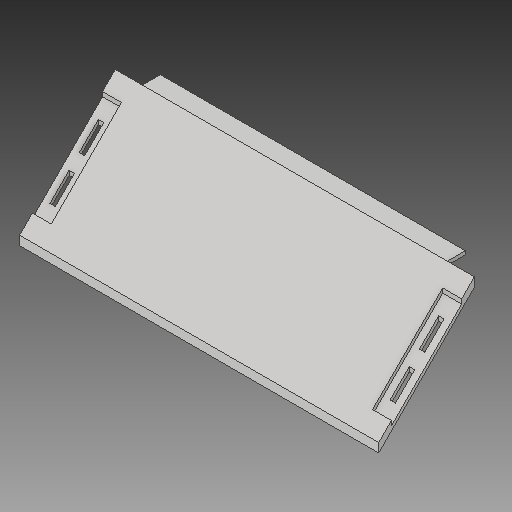
# Autodesk Inventor part: Roof Width Extension
Saved by Autodesk Inventor 2017 (Build 210142000, 142)
## iProperties
Created: 2018-03-29
Part Number: Roof Width Extension
Material: Generic
Document SubType Name: Modeling
Designer: Arjuna
Density: 1 g/cm^3
Appearance: Default
Author: Arjuna
Autodesk Inventor part; units mm, degrees
ref_plane "YZ Plane" through (0, 0, 0) normal (1, 0, 0) x (0, 1, 0)
ref_plane "XZ Plane" through (0, 0, 0) normal (0, 1, 0) x (-1, 0, 0)
ref_plane "XY Plane" through (0, 0, 0) normal (0, 0, 1) x (1, 0, 0)
sketch "Sketch2" plane through (0, 0, 0) normal (0, 0, 1) x (1, 0, 0)
  line L0 (-99.5, 2.5) -> (99.5, 2.5)
  line L1 (99.5, 2.5) -> (99.5, -2.5)
  line L2 (99.5, -2.5) -> (-99.5, -2.5)
  line L3 (-99.5, -2.5) -> (-99.5, 2.5)
  point P0 (0, 0)
  dimension "d1" = 199
  dimension "d2" = 5
  dimension "d3" = 2.5
  dimension "d4" = 99.5
  constraints: 8 end point, 2 parallel, 1 horizontal, 1 perpendicular
  measures "d1" distance of L1.end L2.end
  measures "d2" distance of L2.end L0.start
  measures "d3" vertical distance of point (0, 0) L0.start
  measures "d4" distance from line of point (0, 0) L3
sketch "Sketch3" plane through (0, 0, 0) normal (1, 0, 0) x (0, 1, 0)
  line L0 (0, 0) -> (-53.033, 53.033)
  line L1 (0, -0.5221) -> (1.6531, -0.5221)
  dimension "d5" = 75
  dimension "d6" = 45
  constraints: 4 end point, 1 horizontal
  measures "d5" distance of L0.start L0.end
  measures "d6" angle of L1 L0
sweep "Sweep1" add profiles "Sketch2" path "Sketch3" path curves L0
sketch "Sketch4" plane through (-99.5, 2.5, 0) normal (0, 0.7071068, 0.7071068) x (1, 0, 0)
  line L0 (0, 0) -> (199, 0) projected
  line L1 (0, 0) -> (0, -75) projected
  line L2 (199, -75) -> (0, -75) projected
  line L3 (199, 0) -> (199, -75) projected
  line L4 (199, 0) -> (199, -75)
  line L5 (199, 0) -> (274, -75)
  line L6 (274, -75) -> (199, -75)
  point P0 (99.5, -1.7678)
  dimension "d9" = 45
  constraints: 6 end point, 2 collinear
  measures "d9" angle of L5 L3
sketch "Sketch5" plane through (99.5, -2.5, 0) normal (1, 0, 0) x (0, 0, -1)
  line L0 (0, 5) -> (0, 0) projected
  line L1 (0, 5) -> (-53.033, -48.033) projected
  line L2 (-53.033, -53.033) -> (-53.033, -48.033) projected
  line L3 (0, 0) -> (-53.033, -53.033) projected
  line L4 (-26.5165, -21.5165) -> (-26.5165, -26.5165)
  point P0 (0, 2.5)
  constraints: 2 end point, 2 midpoint
sweep "Sweep2" [suppressed]
mirror "Mirror1" [suppressed]
sketch "Sketch6" plane through (99.5, 2.5, 0) normal (0, 0, -1) x (-1, 0, 0)
  line L0 (199, 0) -> (0, 0) projected
  line L1 (0, 0) -> (0, -5) projected
  line L2 (0, -5) -> (199, -5) projected
  line L3 (199, -5) -> (199, 0) projected
  line L4 (0, 0) -> (199, 0)
  line L5 (199, 0) -> (199, -2)
  line L6 (199, -2) -> (0, -2)
  line L7 (0, -2) -> (0, 0)
  line L8 (98.5, -2) -> (100.5, -2)
  line L9 (100.5, -2) -> (100.5, -5)
  line L10 (100.5, -5) -> (98.5, -5)
  line L11 (98.5, -5) -> (98.5, -2)
  line L12 (48.25, -2) -> (50.25, -2)
  line L13 (50.25, -2) -> (50.25, -5)
  line L14 (50.25, -5) -> (48.25, -5)
  line L15 (48.25, -5) -> (48.25, -2)
  line L16 (148.75, -2) -> (150.75, -2)
  line L17 (150.75, -2) -> (150.75, -5)
  line L18 (150.75, -5) -> (148.75, -5)
  line L19 (148.75, -5) -> (148.75, -2)
  point P0 (99.5, -2.5)
  dimension "d12" = 2
  dimension "d13" = 2
  dimension "d14" = 199
  dimension "d15" = 1
  dimension "d16" = 2
  dimension "d17" = 2
  dimension "d18" = 48.25
  dimension "d19" = 48.25
  dimension "d20" = 48.25
  dimension "d21" = 48.25
  constraints: 32 end point, 8 parallel, 7 point on line, 4 horizontal, 4 perpendicular
  measures "d12" distance between parallel lines of L6 L0
  measures "d13" distance between parallel lines of L9 L11
  measures "d14" distance of L0.start L0.end
  measures "d15" distance from line of L11 point (99.5, -2.5)
  measures "d16" distance of L13.end L14.end
  measures "d17" distance of L17.end L18.end
  measures "d18" distance between parallel lines of L15 L1
  measures "d19" distance between parallel lines of L3 L17
  measures "d20" distance between parallel lines of L11 L13
  measures "d21" distance between parallel lines of L19 L9
extrude "Extrusion1" [suppressed]
sketch "Sketch7" plane through (1, 0.5, 0) normal (0, -1, 0) x (1, 0, 0)
  line L0 (63, 0) -> (63, -10) projected
  line L1 (124, -10) -> (63, -10) projected
  line L2 (124, 0) -> (124, -10) projected
  line L3 (63, 0) -> (124, 0) projected
  line L4 (61, 0) -> (61, -10) projected
  line L5 (0, 0) -> (61, 0) projected
  line L6 (0, 0) -> (0, -10) projected
  line L7 (61, -10) -> (0, -10) projected
  line L8 (-63, 0) -> (-63, -10) projected
  line L9 (-2, -10) -> (-63, -10) projected
  line L10 (-2, 0) -> (-2, -10) projected
  line L11 (-63, 0) -> (-2, 0) projected
  line L12 (-65, -10) -> (-65, 0) projected
  line L13 (-126, 0) -> (-65, 0) projected
  line L14 (-126, 0) -> (-126, -10) projected
  line L15 (-65, -10) -> (-126, -10) projected
  line L16 (67, -4) -> (57, -4)
  line L17 (57, -4) -> (57, -6)
  line L18 (57, -6) -> (67, -6)
  line L19 (67, -6) -> (67, -4)
  line L20 (4, -4) -> (-6, -4)
  line L21 (-6, -4) -> (-6, -6)
  line L22 (-6, -6) -> (4, -6)
  line L23 (4, -6) -> (4, -4)
  line L24 (-59, -4) -> (-69, -4)
  line L25 (-69, -4) -> (-69, -6)
  line L26 (-69, -6) -> (-59, -6)
  line L27 (-59, -6) -> (-59, -4)
  point P0 (-1, 0)
  dimension "d24" = 10
  dimension "d25" = 2
  dimension "d26" = 4
  dimension "d27" = 4
  dimension "d28" = 4
  dimension "d29" = 4
  dimension "d30" = 10
  dimension "d31" = 2
  dimension "d32" = 4
  dimension "d33" = 4
  dimension "d34" = 4
  dimension "d35" = 10
  dimension "d36" = 4
  dimension "d39" = 2
  dimension "d40" = 4
  dimension "d41" = 4
  constraints: 24 end point, 6 parallel, 3 horizontal, 3 perpendicular
  measures "d24" distance of L18.end L17.end
  measures "d25" distance of L16.end L17.end
  measures "d26" distance between parallel lines of L3 L16
  measures "d27" distance between parallel lines of L0 L19
  measures "d28" distance between parallel lines of L17 L4
  measures "d29" distance between parallel lines of L1 L18
  measures "d30" distance of L22.end L21.end
  measures "d31" distance of L20.end L21.end
  measures "d32" distance between parallel lines of L20 L5
  measures "d33" distance between parallel lines of L7 L22
  measures "d34" distance between parallel lines of L6 L23
  measures "d35" distance of L26.end L25.end
  measures "d36" distance between parallel lines of L24 L11
  measures "d39" distance between parallel lines of L26 L24
  measures "d40" distance between parallel lines of L9 L26
  measures "d41" distance between parallel lines of L8 L27
extrude "Extrusion2" [suppressed]
sketch "Sketch10" plane through (99.5, 2.5, 0) normal (0, 0, -1) x (-1, 0, 0)
  line L0 (199, 0) -> (0, 0) projected
  line L1 (0, 0) -> (0, -5) projected
  line L2 (0, -5) -> (199, -5) projected
  line L3 (199, -5) -> (199, 0) projected
  line L4 (15, 0) -> (184, 0)
  line L5 (184, 0) -> (184, -2)
  line L6 (184, -2) -> (15, -2)
  line L7 (15, -2) -> (15, 0)
  point P0 (99.5, -2.5)
  dimension "d76" = 2
  dimension "d77" = 169
  dimension "d78" = 84.5
  constraints: 8 end point, 2 parallel, 1 horizontal, 1 perpendicular, 1 point on line
  measures "d76" distance between parallel lines of L6 L0
  measures "d77" distance between parallel lines of L5 L7
  measures "d78" distance from line of point (99.5, -2.5) L7
extrude "Extrusion5" add sketch "Sketch10" along normal blind 10 contours L5 L6 L7 L0
sketch "Sketch11" plane through (-84.5, 0.5, 0) normal (0, -1, 0) x (1, 0, 0)
  line L0 (0, 0) -> (169, 0) projected
  line L1 (0, 0) -> (0, -10) projected
  line L2 (169, -10) -> (0, -10) projected
  line L3 (169, 0) -> (169, -10) projected
  line L4 (149.25, -6) -> (119.25, -6)
  line L5 (119.25, -6) -> (119.25, -4)
  line L6 (119.25, -4) -> (149.25, -4)
  line L7 (149.25, -4) -> (149.25, -6)
  line L8 (99.5, -6) -> (69.5, -6)
  line L9 (69.5, -6) -> (69.5, -4)
  line L10 (69.5, -4) -> (99.5, -4)
  line L11 (99.5, -4) -> (99.5, -6)
  line L12 (49.75, -6) -> (19.75, -6)
  line L13 (19.75, -6) -> (19.75, -4)
  line L14 (19.75, -4) -> (49.75, -4)
  line L15 (49.75, -4) -> (49.75, -6)
  point P0 (84.5, 0)
  dimension "d81" = 2
  dimension "d82" = 10
  dimension "d83" = 4
  dimension "d84" = 30
  dimension "d85" = 19.75
  dimension "d86" = 169
  dimension "d87" = 19.75
  dimension "d88" = 19.75
  dimension "d89" = 30
  dimension "d90" = 30
  dimension "d91" = 19.75
  constraints: 24 end point, 6 parallel, 4 point on line, 3 horizontal, 3 perpendicular
  measures "d81" distance between parallel lines of L6 L4
  measures "d82" distance of L0.end L2.start
  measures "d83" distance between parallel lines of L0 L6
  measures "d84" distance of L4.start L4.end
  measures "d85" distance between parallel lines of L3 L7
  measures "d86" distance of L2.start L1.end
  measures "d87" distance between parallel lines of L11 L5
  measures "d88" distance between parallel lines of L15 L9
  measures "d89" distance from line of L8.end L11
  measures "d90" distance between parallel lines of L13 L15
  measures "d91" distance between parallel lines of L1 L13
extrude "Extrusion6" add sketch "Sketch11" along normal blind 6 contours L4 L5 L6 L7 | L8 L9 L10 L11 | L12 L13 L14 L15
sketch "Sketch12" plane through (99.5, -2.5, 0) normal (1, 0, 0) x (0, 0, -1)
  line L0 (0, 5) -> (0, 0) projected
  line L1 (0, 5) -> (-53.033, -48.033) projected
  line L2 (-53.033, -53.033) -> (-53.033, -48.033) projected
  line L3 (0, 0) -> (-53.033, -53.033) projected
  line L4 (-7.0711, -2.0711) -> (-7.0711, -4.5711)
  line L5 (-7.0711, -4.5711) -> (-45.9619, -43.4619)
  line L6 (-45.9619, -43.4619) -> (-45.9619, -40.9619)
  line L7 (-45.9619, -40.9619) -> (-7.0711, -2.0711)
  dimension "d99" = 2.5
  dimension "d100" = 10
  dimension "d101" = 10
  constraints: 8 end point, 2 parallel, 2 point on line, 1 collinear, 1 vertical
  measures "d99" distance of L4.start L4.end
  measures "d100" distance of L0.start L4.start
  measures "d101" distance of L1.end L6.end
extrude "Extrusion7" cut sketch "Sketch12" against normal blind 10.5 contours L4 L5 L6 L1
ref_plane "Work Plane1" through (94.25, -2.5, 0) normal (1, 0, 0) x (0, 0, -1)
sketch "Sketch13" plane through (94.25, -2.5, 0) normal (1, 0, 0) x (0, 0, -1)
  line L0 (-7.0711, -2.0711) -> (-7.0711, -4.5711) projected
  line L1 (-7.0711, -4.5711) -> (-45.9619, -43.4619) projected
  line L2 (-45.9619, -43.4619) -> (-45.9619, -40.9619) projected
  line L3 (-45.9619, -40.9619) -> (-53.033, -48.033) projected
  line L4 (-53.033, -53.033) -> (-53.033, -48.033) projected
  line L5 (0, 0) -> (-53.033, -53.033) projected
  line L6 (0, 5) -> (0, 0) projected
  line L7 (0, 5) -> (-7.0711, -2.0711) projected
  line L8 (-45.9619, -40.9619) -> (-7.0711, -2.0711) projected
  line L9 (-45.9619, -43.4619) -> (-45.9619, -40.9619) projected
  line L10 (-7.0711, -4.5711) -> (-45.9619, -43.4619) projected
  line L11 (-7.0711, -2.0711) -> (-7.0711, -4.5711) projected
  line L12 (-13.0815, -10.5815) -> (-13.0815, -13.0815)
  line L13 (-13.0815, -13.0815) -> (-23.6881, -23.6881)
  line L14 (-23.6881, -23.6881) -> (-23.6881, -21.1881)
  line L15 (-23.6881, -21.1881) -> (-13.0815, -10.5815)
  line L16 (-29.3449, -26.8449) -> (-29.3449, -29.3449)
  line L17 (-29.3449, -29.3449) -> (-39.9515, -39.9515)
  line L18 (-39.9515, -39.9515) -> (-39.9515, -37.4515)
  line L19 (-39.9515, -37.4515) -> (-29.3449, -26.8449)
  point P0 (0, 2.5)
  dimension "d104" = 15
  dimension "d105" = 15
  dimension "d106" = 8.5
  dimension "d107" = 8.5
  dimension "d108" = 8
  dimension "d109" = 55
  constraints: 16 end point, 8 point on line, 4 parallel, 1 collinear, 1 vertical
  measures "d104" distance of L16.end L17.end
  measures "d105" distance of L12.end L13.end
  measures "d106" distance of L12.start L0.end
  measures "d107" distance of L18.end L1.end
  measures "d108" distance of L14.end L16.start
  measures "d109" distance of L8.start L8.end
extrude "Extrusion8" cut sketch "Sketch13" along normal mid plane 3 contours L12 L5 L14 L1 | L1 L16 L5 L18
mirror "Mirror2" about plane through (0, 0, 0) normal (1, 0, 0) of "Extrusion7", "Extrusion8"
ref_plane "Work Plane2" through (-94.25, -2.5, 0) normal (1, 0, 0) x (0, 0, -1)
equation "\"d3\" = 0.5 * d2"
equation "\"d4\" = 0.5 * d1"
equation "\"d15\" = 0.5 * d13"
equation "\"d19\" = d18"
equation "\"d30\" = d24"
equation "\"d31\" = d25"
equation "\"d32\" = d26"
equation "\"d34\" = d27"
equation "\"d35\" = d24"
equation "\"d36\" = d26"
equation "\"d39\" = d25"
equation "\"d41\" = d27"
equation "\"d78\" = 0.5 * d77"
equation "\"d83\" = -0.5 * d81 + 0.5 * d82"
equation "\"d85\" = -0.75 * d84 + 0.25 * d86"
equation "\"d87\" = d85"
equation "\"d88\" = d85"
equation "\"d89\" = d84"
equation "\"d90\" = d84"
body "Solid1"
